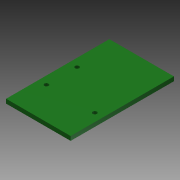
# Autodesk Inventor part: InjectorBoard2
Saved by Autodesk Inventor 2014 (Build 180170000, 170)
## iProperties
Created: 2015-04-18
Part Number: InjectorBoard2
Material: Generic
Document SubType Name: Modeling
Designer: Owner
Density: 1 g/cm^3
Appearance: Smooth - Dark Forest Green
Author: Owner
Autodesk Inventor part; units mm, degrees
ref_plane "YZ Plane" through (0, 0, 0) normal (1, 0, 0) x (0, 1, 0)
ref_plane "XZ Plane" through (0, 0, 0) normal (0, 1, 0) x (-1, 0, 0)
ref_plane "XY Plane" through (0, 0, 0) normal (0, 0, 1) x (1, 0, 0)
sketch "Sketch1" plane through (0, 0, 0) normal (0, 1, 0) x (-1, 0, 0)
  line L0 (-9.3494, 9.1116) -> (16.0506, 9.1116)
  line L1 (16.0506, 9.1116) -> (16.0506, -31.5284)
  line L2 (16.0506, -31.5284) -> (-9.3494, -31.5284)
  line L3 (-9.3494, -31.5284) -> (-9.3494, 9.1116)
  point P0 (0, 0)
  dimension "d0" = 25.4
  dimension "d1" = 40.64
  constraints: 8 end point, 2 parallel, 1 horizontal, 1 perpendicular
  measures "d0" distance of L0.start L0.end
  measures "d1" distance of L0.end L1.end
extrude "Extrusion1" add sketch "Sketch1" along normal blind 1.65
sketch "Sketch2" plane through (0, 1.65, 0) normal (0, 1, 0) x (1, 0, 0)
  line L0 (-16.0506, -9.1116) -> (9.3494, -9.1116) projected
  line L1 (9.3494, -9.1116) -> (9.3494, 31.5284) projected
  line L2 (9.3494, 31.5284) -> (-16.0506, 31.5284) projected
  line L3 (-16.0506, 31.5284) -> (-16.0506, -9.1116) projected
  circle A0 centre (-12.8756, 15.6534) radius 0.7937
  circle A1 centre (-12.8756, 3.5884) radius 0.7937
  circle A2 centre (6.1744, 3.5884) radius 0.7937
  point P0 (0, 0)
  dimension "d4" = 1.5875
  dimension "d5" = 1.5875
  dimension "d6" = 1.5875
  dimension "d7" = 3.175
  dimension "d8" = 3.175
  dimension "d9" = 3.175
  dimension "d10" = 12.7
  dimension "d11" = 12.7
  dimension "d12" = 15.875
  constraints: 3 centre point
  measures "d4" diameter of A2
  measures "d5" diameter of A1
  measures "d6" diameter of A0
  measures "d7" distance from line of L3 A0.centre
  measures "d8" distance from line of L3 A1.centre
  measures "d9" distance from line of L1 A2.centre
  measures "d10" distance from line of L0 A2.centre
  measures "d11" distance from line of L0 A1.centre
  measures "d12" distance from line of L2 A0.centre
extrude "Extrusion2" cut sketch "Sketch2" against normal up to next contours A0 | A1 | A2
body "Solid1"
